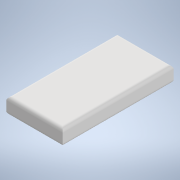
# Autodesk Inventor part: Battery
Saved by Autodesk Inventor 2022 (Build 260153000, 153)
## iProperties
Created: 2020-11-05
Part Number: Battery
Material: Generic
Document SubType Name: Modeling
Designer: simen
Density: 1 g/cm^3
Appearance: Default
Author: simen
Autodesk Inventor part; units mm, degrees
ref_plane "YZ Plane" through (0, 0, 0) normal (1, 0, 0) x (0, 1, 0)
ref_plane "XZ Plane" through (0, 0, 0) normal (0, 1, 0) x (-1, 0, 0)
ref_plane "XY Plane" through (0, 0, 0) normal (0, 0, 1) x (1, 0, 0)
sketch "Sketch1" plane through (0, 0, 0) normal (0, 1, 0) x (-1, 0, 0)
  line L0 (-1464.6959, -2180.3569) -> (-1497.6959, -2180.3569)
  line L1 (-1497.6959, -2180.3569) -> (-1497.6959, -2245.3569)
  line L2 (-1497.6959, -2245.3569) -> (-1464.6959, -2245.3569)
  line L3 (-1464.6959, -2245.3569) -> (-1464.6959, -2180.3569)
  point P0 (0, 0)
  dimension "d0" = 33
  dimension "d1" = 65
  constraints: 8 end point, 2 parallel, 1 horizontal, 1 perpendicular
  measures "d0" distance of L2.end L1.end
  measures "d1" distance of L1.end L0.end
extrude "Extrusion1" add sketch "Sketch1" along normal blind 9.2
fillet "Fillet1" radius 2 8 edges at (1481.1959, 9.2, -2180.3569) (1497.6959, 9.2, -2212.8569) (1497.6959, 0, -2212.8569) (1481.1959, 9.2, -2245.3569) (1464.6959, 9.2, -2212.8569) (1464.6959, 0, -2212.8569) (1481.1959, 0, -2245.3569) (1481.1959, 0, -2180.3569)
body "Solid1"
